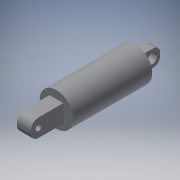
# Autodesk Inventor part: pruzina
Saved by Autodesk Inventor 2016 (Build 200138000, 138)
## iProperties
Created: 2015-06-07
Part Number: pruzina
Material: Generic
Document SubType Name: Modeling
Designer: Jufo
Density: 1 g/cm^3
Appearance: Default
Author: Jufo
Autodesk Inventor part; units mm, degrees
ref_plane "YZ Plane" through (0, 0, 0) normal (1, 0, 0) x (0, 1, 0)
ref_plane "XZ Plane" through (0, 0, 0) normal (0, 1, 0) x (-1, 0, 0)
ref_plane "XY Plane" through (0, 0, 0) normal (0, 0, 1) x (1, 0, 0)
sketch "Sketch1" plane through (0, 0, 0) normal (0, 1, 0) x (-1, 0, 0)
  circle A0 centre (0, 0) radius 8.5
  dimension "d0" = 17
  constraints: 1 centre point, 1 coincident
  measures "d0" diameter of A0
extrude "Extrusion1" add sketch "Sketch1" along normal blind 40
sketch "Sketch2" plane through (0, 40, 0) normal (0, 1, 0) x (1, 0, 0)
  circle A0 centre (0, 0) radius 8.5 projected
  line L0 (0, 0) -> (0, 4.25)
  line L1 (0, 4.25) -> (-2, 4.25)
  line L2 (-2, 4.25) -> (-2, -4.25)
  line L3 (-2, -4.25) -> (2, -4.25)
  line L4 (2, -4.25) -> (2, 4.25)
  line L5 (2, 4.25) -> (0, 4.25)
  dimension "d3" = 4.25
  dimension "d4" = 2
  dimension "d5" = 8.5
  dimension "d6" = 4
  constraints: 12 end point, 3 parallel, 1 collinear, 1 perpendicular, 1 vertical
  measures "d3" distance of L0.start L0.end
  measures "d4" distance of L0.end L1.end
  measures "d5" distance of L1.end L2.end
  measures "d6" distance of L2.end L3.end
extrude "Extrusion2" add sketch "Sketch2" along normal blind 10.6 contours L5 L4 L3 L2 L1
fillet "Fillet1" radius 3.5 2 edges at (0, 50.6, 4.25) (0, 50.6, -4.25)
sketch "Sketch3" plane through (2, 40, 4.25) normal (1, 0, 0) x (0, 0, -1)
  circle A0 centre (4.25, 6.45) radius 2.75
  line L0 (3.5, 10.6) -> (5, 10.6) projected
  point P0 (4.25, -40)
  dimension "d11" = 5.5
  dimension "d26" = 4.15
  constraints: 1 centre point
  measures "d11" diameter of A0
  measures "d26" vertical distance of L0.end A0.centre
extrude "Extrusion3" cut sketch "Sketch3" against normal blind 10.5
sketch "Sketch4" plane through (0, 0, 0) normal (0, -1, 0) x (1, 0, 0)
  circle A0 centre (0, 0) radius 8.5 projected
  line L0 (0, 0) -> (0, 4.5)
  line L1 (0, 4.5) -> (-3, 4.5)
  line L2 (-3, 4.5) -> (-3, -4.5)
  line L3 (-3, -4.5) -> (3, -4.5)
  line L4 (3, -4.5) -> (3, 4.5)
  line L5 (3, 4.5) -> (0, 4.5)
  dimension "d14" = 4.5
  dimension "d15" = 3
  dimension "d16" = 9
  dimension "d17" = 6
  constraints: 12 end point, 3 parallel, 1 collinear, 1 perpendicular, 1 vertical
  measures "d14" distance of L0.start L0.end
  measures "d15" distance of L0.end L1.end
  measures "d16" distance of L1.end L2.end
  measures "d17" distance of L2.end L3.end
extrude "Extrusion4" add sketch "Sketch4" along normal blind 16.6 contours L5 L4 L3 L2 L1
fillet "Fillet2" radius 4 2 edges at (0, -16.6, -4.5) (0, -16.6, 4.5)
sketch "Sketch5" plane through (3, 0, 4.5) normal (1, 0, 0) x (0, 0, -1)
  circle A0 centre (4.5, -12.7) radius 1.5
  line L0 (4, -16.6) -> (5, -16.6) projected
  point P0 (4.5, 0)
  dimension "d22" = 3
  dimension "d27" = 3.9
  constraints: 1 centre point
  measures "d22" diameter of A0
  measures "d27" distance from line of L0 A0.centre
extrude "Extrusion5" cut sketch "Sketch5" against normal blind 16.5
equation "\"d15\" = 0.5 * d17"
body "Solid1"
